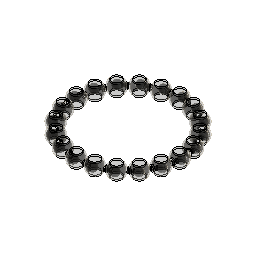
bracelet_design (Autodesk Fusion 360 design; units mm, degrees)
Autodesk Fusion 360 part; units mm, degrees
sphere "SpherePrimitive1" add diameter 10 placed x (1, 0, 0) y (0, 1, 0) z (0, 0, 1) at (0, 0, 0) makes body 1
sphere "SpherePrimitive2" cut diameter 8.5 placed x (1, 0, 0) y (0, 0, -1) z (0, 1, 0) at (0, 0, 0) bodies 1
move_body "Move1" bodies 1 to x (1, 0, 0) y (0, 1, 0) z (0, 0, 1) at (0, -10, 0)
sphere "SpherePrimitive3" add diameter 5 placed x (1, 0, 0) y (0, 1, 0) z (0, 0, 1) at (0, 0, 0) separate body makes body 2
sketch "Sketch4" plane through (0, 0, 0) normal (0, 1, 0) x (1, 0, 0)
  circle A0 centre (0, 0) radius 1
  dimension "d4" = 2
  constraint coincident A0.centre origin
  measures "d4" diameter of A0
extrude "Extrude1" add sketch "Sketch4" against normal blind 5.5 bodies 1 2
fillet "Fillet1" radius 0.5 1 edges at (-0.9323, -2.2913, 0.3616) on bodies 1
fillet "Fillet2" radius 0.5 1 edges at (-0.9323, -5.101, -0.3616) on bodies 1
move_body "Move2" bodies 1 to x (1, 0, 0) y (0, 1, 0) z (0, 0, 1) at (0, 10, 0)
sketch "Sketch5" plane through (0, 0, 0) normal (0, 1, 0) x (1, 0, 0)
  circle A0 centre (0, 0) radius 1.75
  dimension "d11" = 3.5
  constraint coincident A0.centre origin
  measures "d11" diameter of A0
extrude "Extrude2" cut sketch "Sketch5" against normal blind 8 bodies 1
sketch "Sketch6" plane through (0, 0, 0) normal (1, 0, 0) x (0, 1, 0)
  circle A0 centre (0, 0) radius 3
  dimension "d14" = 6
  constraint coincident A0.centre origin
  measures "d14" diameter of A0
extrude "Extrude3" cut sketch "Sketch6" along normal blind 7 bodies 1
extrude "Extrude4" cut sketch "Sketch6" against normal blind 7.5 bodies 1
sketch "Sketch8" plane through (0, 0, 0) normal (0, 0, 1) x (1, 0, 0)
  circle A0 centre (0, 0) radius 30
  constraint coincident A0.centre origin
move_body "Move5" bodies 1 to x (1, 0, 0) y (0, 1, 0) z (0, 0, 1) at (30, 0, 0)
move_body "Move6" bodies 1 to x (0, 0, -1) y (0, 1, 0) z (1, 0, 0) at (30, 0, 30)
sketch "Sketch10" plane through (0, 0, 0) normal (0, 0, 1) x (1, 0, 0)
  circle A0 centre (0, 0) radius 33
  dimension "d24" = 66
  constraint coincident A0.centre origin
  measures "d24" diameter of A0
move_body "Move11" bodies 1 to x (1, 0, 0) y (0, 1, 0) z (0, 0, 1) at (3, 0, 0)
move_body "Move12" bodies 1 to x (1, 0, 0) y (0, 1, 0) z (0, 0, 1) at (-1, 0, 0)
pattern_circular "C-Pattern3" count 20 over 360 about axis through (0, 0, 0) along (0, 0, 1) of bodies 1 makes body 3 at (28.1312, 13.7706, 2.1512) makes body 4 at (22.499, 21.7897, 2.1512) makes body 5 at (14.6645, 27.6758, 2.1512) makes body 6 at (5.3945, 30.8528, 2.1512) makes body 7 at (-4.4036, 31.0097, 2.1512) makes body 8 at (-13.7706, 28.1312, 2.1512) makes body 9 at (-21.7897, 22.499, 2.1512) makes body 10 at (-27.6758, 14.6645, 2.1512) makes body 11 at (-30.8528, 5.3945, 2.1512) makes body 12 at (-31.0097, -4.4036, 2.1512) makes body 13 at (-28.1312, -13.7706, 2.1512) makes body 14 at (-22.499, -21.7897, 2.1512) makes body 15 at (-14.6645, -27.6758, 2.1512) makes body 16 at (-5.3945, -30.8528, 2.1512) makes body 17 at (4.4036, -31.0097, 2.1512) makes body 18 at (13.7706, -28.1312, 2.1512) makes body 19 at (21.7897, -22.499, 2.1512) makes body 20 at (27.6758, -14.6645, 2.1512) makes body 21 at (30.8528, -5.3945, 2.1512)
